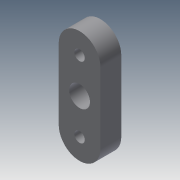
# Autodesk Inventor part: gearSupport
Saved by Autodesk Inventor 2015 (Build 190159000, 159)
## iProperties
Created: 2014-08-31
Part Number: gearSupport
Material: Generic
Document SubType Name: Modeling
Designer: shohei
Density: 1 g/cm^3
Appearance: Default
Author: shohei
Autodesk Inventor part; units mm, degrees
ref_plane "YZ Plane" through (0, 0, 0) normal (1, 0, 0) x (0, 1, 0)
ref_plane "XZ Plane" through (0, 0, 0) normal (0, 1, 0) x (-1, 0, 0)
ref_plane "XY Plane" through (0, 0, 0) normal (0, 0, 1) x (1, 0, 0)
sketch "Block1" plane through (0, 0, 0) normal (0, 0, 1) x (1, 0, 0)
  circle A0 centre (0, 0) radius 20.22
  circle A1 centre (0, 12) radius 2.72
  circle A2 centre (0, 0) radius 5.22
  circle A3 centre (0, -12) radius 2.72
sketch "Block2" plane through (0, 0, 0) normal (0, 0, 1) x (1, 0, 0)
  circle A0 centre (0, 0) radius 22.72
  circle A1 centre (-12, 12) radius 2.72
  circle A2 centre (0, 0) radius 5.22
  point P0 (-4, 4)
sketch "Sketch9" plane through (0, 0, 0) normal (0, 1, 0) x (-1, 0, 0)
  line L0 (0, -16.9706) -> (0, 16.9706) construction
  line L1 (10, -16.9706) -> (10, 16.9706)
  line L2 (-10, 16.9706) -> (-10, -16.9706)
  arc A0 (-10, -16.9706) -> (10, -16.9706) centre (0, -16.9706) ccw
  arc A1 (10, 16.9706) -> (-10, 16.9706) centre (0, 16.9706) ccw
  circle A2 centre (0, 0) radius 5
  circle A3 centre (0, 16.9706) radius 2.5
  circle A4 centre (0, -16.9706) radius 2.5
  dimension "d33" = 10
  dimension "d34" = 33.9411
  dimension "d35" = 10
  dimension "d36" = 5
  dimension "d37" = 5
  constraints: 8 end point, 5 centre point, 4 point on circle, 4 tangent, 3 coincident, 1 midpoint, 1 parallel, 1 vertical
  measures "d33" radius of A1
  measures "d34" distance of L1.start L1.end
  measures "d35" diameter of A2
  measures "d36" diameter of A3
  measures "d37" diameter of A4
extrude "Extrusion6" add sketch "Sketch9" along normal blind 10
body "Solid4"
